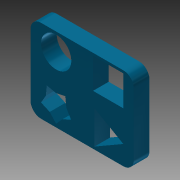
# Autodesk Inventor part: Passenger Base
Saved by Autodesk Inventor 2015 (Build 190159000, 159)
## iProperties
Created: 2014-10-30
Part Number: Passenger Base
Material: Generic
Document SubType Name: Modeling
Designer: ahall212
Density: 1 g/cm^3
Appearance: Sky Blue Dark
Author: ahall212
Autodesk Inventor part; units mm, degrees
ref_plane "YZ Plane" through (0, 0, 0) normal (1, 0, 0) x (0, 1, 0)
ref_plane "XZ Plane" through (0, 0, 0) normal (0, 1, 0) x (-1, 0, 0)
ref_plane "XY Plane" through (0, 0, 0) normal (0, 0, 1) x (1, 0, 0)
sketch "Sketch1" plane through (0, 0, 0) normal (0, 0, 1) x (1, 0, 0)
  line L0 (5.08, 0) -> (45.085, 0)
  line L1 (50.165, 5.08) -> (50.165, 35.306)
  line L2 (45.085, 40.386) -> (5.08, 40.386)
  line L3 (0, 35.306) -> (0, 5.08)
  arc A0 (5.08, 40.386) -> (0, 35.306) centre (5.08, 35.306) ccw
  arc A1 (0, 5.08) -> (5.08, 0) centre (5.08, 5.08) ccw
  arc A2 (45.085, 0) -> (50.165, 5.08) centre (45.085, 5.08) ccw
  arc A3 (50.165, 35.306) -> (45.085, 40.386) centre (45.085, 35.306) ccw
  point P0 (0, 0)
  point P1 (50.165, 0)
  point P2 (50.165, 40.386)
  point P3 (0, 40.386)
  dimension "d0" = 50.165
  dimension "d1" = 40.386
  dimension "d2" = 5.08
  constraints: 8 end point, 8 point on circle, 8 point on line, 8 tangent, 4 centre point, 3 equal radius, 3 perpendicular, 1 horizontal
  measures "d0" distance of point (50.165, 40.386) point (0, 40.386)
  measures "d1" distance of point (50.165, 0) point (50.165, 40.386)
  measures "d2" radius of A0
extrude "Extrusion1" add sketch "Sketch1" along normal blind 7.62
sketch "Sketch2" plane through (0, 0, 7.62) normal (0, 0, 1) x (1, 0, 0)
  circle A0 centre (12.446, 31.75) radius 7.366
  line L0 (45.085, 40.386) -> (5.08, 40.386) projected
  line L1 (0, 35.306) -> (0, 5.08) projected
  line L2 (30.353, 39.116) -> (45.085, 39.116)
  line L3 (45.085, 39.116) -> (45.085, 24.384)
  line L4 (45.085, 24.384) -> (30.353, 24.384)
  line L5 (30.353, 24.384) -> (30.353, 39.116)
  line L6 (50.165, 5.08) -> (50.165, 35.306) projected
  line L7 (31.0509, 17.4752) -> (31.0509, 1.27)
  line L8 (31.0509, 1.27) -> (45.085, 9.3726)
  line L9 (45.085, 9.3726) -> (31.0509, 17.4752)
  line L10 (5.08, 0) -> (45.085, 0) projected
  circle A1 centre (12.3952, 9.2202) radius 7.6835
  circle A2 centre (12.3952, 9.2202) radius 5.2324
  line L11 (12.3952, 1.5367) -> (5.0878, 6.8459)
  line L12 (5.0878, 6.8459) -> (7.879, 15.4363)
  line L13 (7.879, 15.4363) -> (16.9114, 15.4363)
  line L14 (16.9114, 15.4363) -> (19.7026, 6.8459)
  line L15 (19.7026, 6.8459) -> (12.3952, 1.5367)
  line L16 (7.879, 15.4363) -> (12.3952, 14.4526)
  line L17 (12.3952, 14.4526) -> (16.9114, 15.4363)
  line L18 (16.9114, 15.4363) -> (17.3715, 10.8371)
  line L19 (17.3715, 10.8371) -> (19.7026, 6.8459)
  line L20 (12.3952, 1.5367) -> (15.4707, 4.9871)
  line L21 (15.4707, 4.9871) -> (19.7026, 6.8459)
  line L22 (12.3952, 1.5367) -> (9.3197, 4.9871)
  line L23 (9.3197, 4.9871) -> (5.0878, 6.8459)
  line L24 (5.0878, 6.8459) -> (7.4189, 10.8371)
  line L25 (7.4189, 10.8371) -> (7.879, 15.4363)
  point P0 (0, 0)
  dimension "d16" = 15.367
  dimension "d5" = 14.732
  dimension "d6" = 8.636
  dimension "d7" = 12.446
  dimension "d8" = 14.732
  dimension "d9" = 14.732
  dimension "d10" = 5.08
  dimension "d11" = 1.27
  dimension "d12" = 16.2052
  dimension "d13" = 5.08
  dimension "d14" = 1.27
  dimension "d17" = 10.4648
  dimension "d18" = 12.3952
  dimension "d19" = 9.2202
  constraints: 44 end point, 7 equal length, 5 point on circle, 2 centre point, 2 coincident, 2 parallel, 1 horizontal, 1 perpendicular, 1 vertical, 1 vertical alignment, 13 other
  measures "d5" diameter of A0
  measures "d6" distance from line of L0 A0.centre
  measures "d7" distance from line of L1 A0.centre
  measures "d8" distance of L3.end L4.end
  measures "d9" distance of L2.end L3.end
  measures "d10" distance between parallel lines of L6 L3
  measures "d11" distance between parallel lines of L0 L2
  measures "d12" distance of L7.start L7.end
  measures "d13" distance from line of L6 L8.end
  measures "d14" distance from line of L10 L7.end
  measures "d17" diameter of A2
  measures "d18" distance from line of L1 point (12.395, 9.22)
  measures "d19" distance from line of L10 point (12.395, 9.22)
extrude "Extrusion2" cut sketch "Sketch2" against normal through all contours A0 | L2 L3 L4 L5 | L9 L8 L7 | L18 A2 L17 | L21 A2 L19 | L16 A2 L25 | A2 | L22 A2 L20 | L24 A2 L23
shell "Shell1" thickness 2.54 removed faces 1 at (40.407, 17.0773, 0)
body "Solid1"
